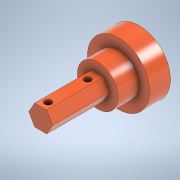
# Autodesk Inventor part: jigForHexBushingForConnectorPiece
Saved by Autodesk Inventor 2022.1 (Build 261234000, 234)
## iProperties
Created: 2020-11-16
Part Number: jigForHexBushingForConnectorPiece
Material: PC/ABS Plastic
Document SubType Name: Modeling
Designer: robst
Density: 0.357273 g/cm^3
Appearance: Smooth - Light Orange
Author: robst
Autodesk Inventor part; units mm, degrees
ref_plane "YZ Plane" through (0, 0, 0) normal (1, 0, 0) x (0, 1, 0)
ref_plane "XZ Plane" through (0, 0, 0) normal (0, 1, 0) x (-1, 0, 0)
ref_plane "XY Plane" through (0, 0, 0) normal (0, 0, 1) x (1, 0, 0)
sketch "Sketch1" plane through (0, 0, 0) normal (0, 0, 1) x (1, 0, 0)
  line L0 (7.3323, 0) -> (3.6662, -6.35)
  line L1 (3.6662, -6.35) -> (-3.6662, -6.35)
  line L2 (-3.6662, -6.35) -> (-7.3323, 0)
  line L3 (-7.3323, 0) -> (-3.6662, 6.35)
  line L4 (-3.6662, 6.35) -> (3.6662, 6.35)
  line L5 (3.6662, 6.35) -> (7.3323, 0)
  point P0 (0, 0)
  point P1 (0, 0)
  dimension "d0" = 12.7
  constraints: 12 end point, 1 coincident, 1 horizontal, 13 other
  measures "d0" distance between parallel lines of L1 L4
extrude "Extrusion1" add sketch "Sketch1" along normal mid plane 34.925
sketch "Sketch2" plane through (0, 0, -17.4625) normal (0, 0, -1) x (-1, 0, 0)
  circle A0 centre (0, 0) radius 12.5095
  dimension "d3" = 25.019
  constraints: 1 centre point, 1 coincident
  measures "d3" diameter of A0
extrude "Extrusion2" add sketch "Sketch2" along normal blind 12.7
sketch "Sketch3" plane through (0, 0, -30.1625) normal (0, 0, -1) x (-1, 0, 0)
  circle A0 centre (0, 0) radius 19.05
  dimension "d6" = 38.1
  constraints: 1 centre point, 1 coincident
  measures "d6" diameter of A0
extrude "Extrusion3" add sketch "Sketch3" along normal blind 12.7
sketch "Sketch4" plane through (0, 0, -42.8625) normal (0, 0, -1) x (-1, 0, 0)
  circle A0 centre (0, 0) radius 16.51 construction
  line L0 (-14.4198, 2.5806) -> (-14.4677, 2.1014)
  line L1 (-14.4677, 2.1014) -> (-16.0898, 2.2636)
  spline S0 degree 2 poles (-16.0898, 2.2636) (-16.2865, 2.2832) (-16.6281, 2.2802) (-16.735, 2.235) knots 0 0 0 1 2 2 2
  spline S1 degree 2 poles (-16.735, 2.235) (-16.8484, 2.1874) (-16.9737, 1.9889) (-16.9915, 1.8107) knots 0 0 0 1 2 2 2
  spline S2 degree 2 poles (-16.9915, 1.8107) (-17.0093, 1.6325) (-16.8566, 1.2356) (-16.7212, 1.039) knots 0 0 0 1 2 2 2
  line L2 (-16.7212, 1.039) -> (-14.5952, 0.8264)
  line L3 (-14.5952, 0.8264) -> (-14.6431, 0.3472)
  line L4 (-14.6431, 0.3472) -> (-18.6032, 0.7431)
  line L5 (-18.6032, 0.7431) -> (-18.5553, 1.2224)
  line L6 (-18.5553, 1.2224) -> (-17.1236, 1.0792)
  spline S3 degree 2 poles (-17.1236, 1.0792) (-17.2957, 1.3137) (-17.457, 1.7487) (-17.4336, 1.9822) knots 0 0 0 1 2 2 2
  spline S4 degree 2 poles (-17.4336, 1.9822) (-17.3918, 2.4) (-16.7915, 2.8178) (-16.2662, 2.7653) knots 0 0 0 1 2 2 2
  line L7 (-16.2662, 2.7653) -> (-14.4198, 2.5806)
  spline S5 degree 2 poles (-13.8575, 4.4081) (-14.0557, 3.752) (-15.0096, 3.2532) (-15.6893, 3.4586) knots 0 0 0 1 2 2 2
  spline S6 degree 2 poles (-15.6893, 3.4586) (-16.3573, 3.6604) (-16.9377, 4.6002) (-16.7672, 5.1647) knots 0 0 0 1 2 2 2
  spline S7 degree 2 poles (-16.7672, 5.1647) (-16.6904, 5.4189) (-16.4238, 5.7673) (-16.2234, 5.8648) knots 0 0 0 1 2 2 2
  spline S8 degree 2 poles (-16.2234, 5.8648) (-16.0221, 5.9653) (-15.5226, 5.9853) (-15.1945, 5.8861) knots 0 0 0 1 2 2 2
  line L8 (-15.1945, 5.8861) -> (-14.9433, 5.8102)
  line L9 (-14.9433, 5.8102) -> (-15.5157, 3.9157)
  spline S9 degree 2 poles (-15.5157, 3.9157) (-15.0399, 3.7719) (-14.3898, 4.098) (-14.2612, 4.5236) knots 0 0 0 1 2 2 2
  spline S10 degree 2 poles (-14.2612, 4.5236) (-14.2157, 4.6744) (-14.1952, 4.9875) (-14.2127, 5.1218) knots 0 0 0 1 2 2 2
  spline S11 degree 2 poles (-14.2127, 5.1218) (-14.2343, 5.2638) (-14.286, 5.4665) (-14.3163, 5.5369) knots 0 0 0 1 2 2 2
  line L10 (-14.3163, 5.5369) -> (-14.3083, 5.5635)
  line L11 (-14.3083, 5.5635) -> (-13.8058, 5.4117)
  spline S12 degree 2 poles (-13.8058, 5.4117) (-13.7974, 5.3221) (-13.7761, 5.0511) (-13.778, 4.9485) knots 0 0 0 1 2 2 2
  spline S13 degree 2 poles (-13.778, 4.9485) (-13.7798, 4.8039) (-13.8075, 4.5736) (-13.8575, 4.4081) knots 0 0 0 1 2 2 2
  spline S14 degree 2 poles (-15.4307, 5.4673) (-15.6187, 5.5176) (-15.9139, 5.5229) (-16.0278, 5.4767) knots 0 0 0 1 2 2 2
  spline S15 degree 2 poles (-16.0278, 5.4767) (-16.1554, 5.4282) (-16.3406, 5.21) (-16.3969, 5.0238) knots 0 0 0 1 2 2 2
  spline S16 degree 2 poles (-16.3969, 5.0238) (-16.4523, 4.8406) (-16.4206, 4.5504) (-16.3464, 4.4118) knots 0 0 0 1 2 2 2
  spline S17 degree 2 poles (-16.3464, 4.4118) (-16.2683, 4.2753) (-16.0374, 4.0895) (-15.8674, 4.022) knots 0 0 0 1 2 2 2
  line L12 (-15.8674, 4.022) -> (-15.4307, 5.4673)
  line L13 (-12.3977, 7.8243) -> (-12.668, 7.3002)
  line L14 (-12.668, 7.3002) -> (-13.9414, 7.1752)
  line L15 (-13.9414, 7.1752) -> (-13.3133, 6.0489)
  line L16 (-13.3133, 6.0489) -> (-13.5637, 5.5632)
  line L17 (-13.5637, 5.5632) -> (-14.3691, 7.0936)
  line L18 (-14.3691, 7.0936) -> (-16.1006, 6.8818)
  line L19 (-16.1006, 6.8818) -> (-15.8303, 7.4059)
  line L20 (-15.8303, 7.4059) -> (-14.5666, 7.5324)
  line L21 (-14.5666, 7.5324) -> (-15.1893, 8.649)
  line L22 (-15.1893, 8.649) -> (-14.9388, 9.1347)
  line L23 (-14.9388, 9.1347) -> (-14.1361, 7.6126)
  line L24 (-14.1361, 7.6126) -> (-12.3977, 7.8243)
  spline S18 degree 2 poles (-11.4795, 10.9139) (-11.2568, 10.7375) (-11.0498, 10.2978) (-11.0496, 10.0692) knots 0 0 0 1 2 2 2
  spline S19 degree 2 poles (-11.0496, 10.0692) (-11.0532, 9.7963) (-11.2467, 9.3233) (-11.4882, 9.0183) knots 0 0 0 1 2 2 2
  line L25 (-11.4882, 9.0183) -> (-12.167, 8.1616)
  line L26 (-12.167, 8.1616) -> (-15.1534, 10.5275)
  line L27 (-15.1534, 10.5275) -> (-14.5264, 11.3189)
  spline S20 degree 2 poles (-14.5264, 11.3189) (-14.2734, 11.6383) (-13.9792, 11.9252) (-13.7843, 12.0071) knots 0 0 0 1 2 2 2
  spline S21 degree 2 poles (-13.7843, 12.0071) (-13.5711, 12.1022) (-13.1758, 12.0293) (-12.9871, 11.8798) knots 0 0 0 1 2 2 2
  spline S22 degree 2 poles (-12.9871, 11.8798) (-12.7765, 11.713) (-12.6189, 11.2257) (-12.6798, 10.9549) knots 0 0 0 1 2 2 2
  line L28 (-12.6798, 10.9549) -> (-12.6653, 10.9434)
  spline S23 degree 2 poles (-12.6653, 10.9434) (-12.3818, 11.1521) (-11.765, 11.1401) (-11.4795, 10.9139) knots 0 0 0 1 2 2 2
  spline S24 degree 2 poles (-11.7904, 10.4866) (-11.9598, 10.6208) (-12.2543, 10.6966) (-12.4467, 10.6127) knots 0 0 0 1 2 2 2
  spline S25 degree 2 poles (-12.4467, 10.6127) (-12.5699, 10.5567) (-12.7753, 10.357) (-12.9383, 10.1513) knots 0 0 0 1 2 2 2
  line L29 (-12.9383, 10.1513) -> (-13.2949, 9.7012)
  line L30 (-13.2949, 9.7012) -> (-12.1913, 8.8269)
  line L31 (-12.1913, 8.8269) -> (-11.9363, 9.1488)
  spline S26 degree 2 poles (-11.9363, 9.1488) (-11.7293, 9.4102) (-11.54, 9.7486) (-11.5254, 9.9261) knots 0 0 0 1 2 2 2
  spline S27 degree 2 poles (-11.5254, 9.9261) (-11.517, 10.1007) (-11.6331, 10.362) (-11.7904, 10.4866) knots 0 0 0 1 2 2 2
  spline S28 degree 2 poles (-13.2592, 11.4218) (-13.3657, 11.5062) (-13.583, 11.5601) (-13.6922, 11.5167) knots 0 0 0 1 2 2 2
  spline S29 degree 2 poles (-13.6922, 11.5167) (-13.8222, 11.4621) (-14.0323, 11.2465) (-14.1991, 11.0359) knots 0 0 0 1 2 2 2
  line L32 (-14.1991, 11.0359) -> (-14.5001, 10.656)
  line L33 (-14.5001, 10.656) -> (-13.6265, 9.9638)
  line L34 (-13.6265, 9.9638) -> (-13.2699, 10.414)
  spline S30 degree 2 poles (-13.2699, 10.414) (-13.1222, 10.6003) (-13.021, 10.8077) (-13.0067, 10.95) knots 0 0 0 1 2 2 2
  spline S31 degree 2 poles (-13.0067, 10.95) (-12.992, 11.088) (-13.1189, 11.3106) (-13.2592, 11.4218) knots 0 0 0 1 2 2 2
  line L35 (-8.5093, 11.9219) -> (-8.879, 11.6132)
  line L36 (-8.879, 11.6132) -> (-9.0809, 11.8549)
  spline S32 degree 2 poles (-9.0809, 11.8549) (-9.1268, 11.5631) (-9.3038, 11.1537) (-9.4934, 10.9954) knots 0 0 0 1 2 2 2
  spline S33 degree 2 poles (-9.4934, 10.9954) (-9.6356, 10.8767) (-9.9683, 10.7597) (-10.1459, 10.7844) knots 0 0 0 1 2 2 2
  spline S34 degree 2 poles (-10.1459, 10.7844) (-10.3257, 10.8071) (-10.6893, 11.0304) (-10.8753, 11.2532) knots 0 0 0 1 2 2 2
  line L37 (-10.8753, 11.2532) -> (-12.0649, 12.6774)
  line L38 (-12.0649, 12.6774) -> (-11.6952, 12.9861)
  line L39 (-11.6952, 12.9861) -> (-10.6502, 11.7349)
  spline S35 degree 2 poles (-10.6502, 11.7349) (-10.5037, 11.5596) (-10.2856, 11.3515) (-10.1694, 11.3038) knots 0 0 0 1 2 2 2
  spline S36 degree 2 poles (-10.1694, 11.3038) (-10.0531, 11.2561) (-9.8337, 11.3065) (-9.6892, 11.4273) knots 0 0 0 1 2 2 2
  spline S37 degree 2 poles (-9.6892, 11.4273) (-9.5541, 11.5401) (-9.3771, 11.9494) (-9.3421, 12.1677) knots 0 0 0 1 2 2 2
  line L40 (-9.3421, 12.1677) -> (-10.7118, 13.8075)
  line L41 (-10.7118, 13.8075) -> (-10.3421, 14.1163)
  line L42 (-10.3421, 14.1163) -> (-8.5093, 11.9219)
  spline S38 degree 2 poles (-7.2187, 12.6182) (-7.4684, 12.4765) (-7.9769, 12.3653) (-8.1619, 12.3597) knots 0 0 0 1 2 2 2
  line L43 (-8.1619, 12.3597) -> (-8.4286, 12.8296)
  line L44 (-8.4286, 12.8296) -> (-8.4071, 12.8417)
  spline S39 degree 2 poles (-8.4071, 12.8417) (-8.3291, 12.8293) (-8.1261, 12.8096) (-7.9733, 12.8218) knots 0 0 0 1 2 2 2
  spline S40 degree 2 poles (-7.9733, 12.8218) (-7.8396, 12.8302) (-7.5392, 12.9014) (-7.4023, 12.9791) knots 0 0 0 1 2 2 2
  spline S41 degree 2 poles (-7.4023, 12.9791) (-7.3029, 13.0355) (-7.1006, 13.2107) (-7.0682, 13.2788) knots 0 0 0 1 2 2 2
  spline S42 degree 2 poles (-7.0682, 13.2788) (-7.0193, 13.374) (-7.0151, 13.5291) (-7.0821, 13.6472) knots 0 0 0 1 2 2 2
  spline S43 degree 2 poles (-7.0821, 13.6472) (-7.166, 13.7949) (-7.414, 13.8565) (-7.6497, 13.7901) knots 0 0 0 1 2 2 2
  spline S44 degree 2 poles (-7.6497, 13.7901) (-7.7409, 13.7632) (-8.0291, 13.6706) (-8.156, 13.6376) knots 0 0 0 1 2 2 2
  spline S45 degree 2 poles (-8.156, 13.6376) (-8.4879, 13.5593) (-8.9407, 13.7566) (-9.0794, 14.0009) knots 0 0 0 1 2 2 2
  spline S46 degree 2 poles (-9.0794, 14.0009) (-9.2715, 14.3392) (-9.0034, 15.0489) (-8.5845, 15.2867) knots 0 0 0 1 2 2 2
  spline S47 degree 2 poles (-8.5845, 15.2867) (-8.3778, 15.4041) (-7.901, 15.5398) (-7.7145, 15.5428) knots 0 0 0 1 2 2 2
  line L45 (-7.7145, 15.5428) -> (-7.4599, 15.0944)
  line L46 (-7.4599, 15.0944) -> (-7.4814, 15.0822)
  spline S48 degree 2 poles (-7.4814, 15.0822) (-7.7157, 15.1196) (-8.1915, 15.0447) (-8.3929, 14.9304) knots 0 0 0 1 2 2 2
  spline S49 degree 2 poles (-8.3929, 14.9304) (-8.5996, 14.813) (-8.7852, 14.4769) (-8.6861, 14.3024) knots 0 0 0 1 2 2 2
  spline S50 degree 2 poles (-8.6861, 14.3024) (-8.5961, 14.144) (-8.3401, 14.087) (-8.1247, 14.1453) knots 0 0 0 1 2 2 2
  spline S51 degree 2 poles (-8.1247, 14.1453) (-8.0197, 14.173) (-7.7613, 14.2557) (-7.6184, 14.2979) knots 0 0 0 1 2 2 2
  spline S52 degree 2 poles (-7.6184, 14.2979) (-7.3049, 14.3835) (-6.8442, 14.2225) (-6.6872, 13.946) knots 0 0 0 1 2 2 2
  spline S53 degree 2 poles (-6.6872, 13.946) (-6.5958, 13.7849) (-6.5604, 13.4286) (-6.6245, 13.2538) knots 0 0 0 1 2 2 2
  spline S54 degree 2 poles (-6.6245, 13.2538) (-6.6935, 13.069) (-6.9636, 12.763) (-7.2187, 12.6182) knots 0 0 0 1 2 2 2
  line L47 (-3.7576, 14.1588) -> (-4.2122, 13.9996)
  line L48 (-4.2122, 13.9996) -> (-4.751, 15.5382)
  spline S55 degree 2 poles (-4.751, 15.5382) (-4.8163, 15.7247) (-4.9635, 16.033) (-5.0496, 16.1108) knots 0 0 0 1 2 2 2
  spline S56 degree 2 poles (-5.0496, 16.1108) (-5.1407, 16.1934) (-5.3736, 16.223) (-5.5426, 16.1639) knots 0 0 0 1 2 2 2
  spline S57 degree 2 poles (-5.5426, 16.1639) (-5.7116, 16.1047) (-6.0068, 15.7985) (-6.1277, 15.5926) knots 0 0 0 1 2 2 2
  line L49 (-6.1277, 15.5926) -> (-5.4215, 13.5761)
  line L50 (-5.4215, 13.5761) -> (-5.8761, 13.4169)
  line L51 (-5.8761, 13.4169) -> (-7.1915, 17.1731)
  line L52 (-7.1915, 17.1731) -> (-6.7369, 17.3322)
  line L53 (-6.7369, 17.3322) -> (-6.2613, 15.9743)
  spline S58 degree 2 poles (-6.2613, 15.9743) (-6.1216, 16.2293) (-5.7956, 16.5594) (-5.5741, 16.637) knots 0 0 0 1 2 2 2
  spline S59 degree 2 poles (-5.5741, 16.637) (-5.1778, 16.7757) (-4.5454, 16.4084) (-4.3709, 15.9101) knots 0 0 0 1 2 2 2
  line L54 (-4.3709, 15.9101) -> (-3.7576, 14.1588)
  line L55 (-2.6108, 14.3718) -> (-3.0832, 14.2779)
  line L56 (-3.0832, 14.2779) -> (-3.6405, 17.0821)
  line L57 (-3.6405, 17.0821) -> (-3.1681, 17.176)
  line L58 (-3.1681, 17.176) -> (-2.6108, 14.3718)
  line L59 (-3.2275, 17.6489) -> (-3.7635, 17.5424)
  line L60 (-3.7635, 17.5424) -> (-3.861, 18.033)
  line L61 (-3.861, 18.033) -> (-3.325, 18.1395)
  line L62 (-3.325, 18.1395) -> (-3.2275, 17.6489)
  line L63 (0.3206, 14.6454) -> (-0.1603, 14.6186)
  line L64 (-0.1603, 14.6186) -> (-0.2508, 16.2463)
  spline S60 degree 2 poles (-0.2508, 16.2463) (-0.2617, 16.4436) (-0.3176, 16.7807) (-0.3787, 16.8793) knots 0 0 0 1 2 2 2
  spline S61 degree 2 poles (-0.3787, 16.8793) (-0.4433, 16.984) (-0.6588, 17.0771) (-0.8376, 17.0672) knots 0 0 0 1 2 2 2
  spline S62 degree 2 poles (-0.8376, 17.0672) (-1.0164, 17.0572) (-1.3849, 16.845) (-1.5582, 16.6808) knots 0 0 0 1 2 2 2
  line L65 (-1.5582, 16.6808) -> (-1.4396, 14.5475)
  line L66 (-1.4396, 14.5475) -> (-1.9205, 14.5208)
  line L67 (-1.9205, 14.5208) -> (-2.0792, 17.3754)
  line L68 (-2.0792, 17.3754) -> (-1.5983, 17.4022)
  line L69 (-1.5983, 17.4022) -> (-1.5807, 17.0846)
  spline S63 degree 2 poles (-1.5807, 17.0846) (-1.3757, 17.2908) (-0.9708, 17.5174) (-0.7365, 17.5305) knots 0 0 0 1 2 2 2
  spline S64 degree 2 poles (-0.7365, 17.5305) (-0.3173, 17.5538) (0.1883, 17.0253) (0.2176, 16.4981) knots 0 0 0 1 2 2 2
  line L70 (0.2176, 16.4981) -> (0.3206, 14.6454)
  spline S65 degree 2 poles (1.0284, 14.1458) (1.0743, 14.1174) (1.251, 14.0233) (1.3662, 13.9787) knots 0 0 0 1 2 2 2
  spline S66 degree 2 poles (1.3662, 13.9787) (1.4928, 13.9261) (1.7102, 13.8543) (1.8416, 13.8354) knots 0 0 0 1 2 2 2
  spline S67 degree 2 poles (1.8416, 13.8354) (2.0616, 13.8037) (2.3839, 13.8759) (2.4844, 13.9674) knots 0 0 0 1 2 2 2
  spline S68 degree 2 poles (2.4844, 13.9674) (2.5819, 14.0595) (2.6852, 14.3222) (2.7103, 14.4964) knots 0 0 0 1 2 2 2
  line L71 (2.7103, 14.4964) -> (2.7459, 14.744)
  spline S69 degree 2 poles (2.7459, 14.744) (2.5292, 14.6036) (2.1366, 14.4979) (1.8585, 14.5379) knots 0 0 0 1 2 2 2
  spline S70 degree 2 poles (1.8585, 14.5379) (1.3756, 14.6074) (0.9075, 15.4078) (1.0047, 16.0832) knots 0 0 0 1 2 2 2
  spline S71 degree 2 poles (1.0047, 16.0832) (1.0553, 16.4347) (1.3322, 16.95) (1.525, 17.1188) knots 0 0 0 1 2 2 2
  spline S72 degree 2 poles (1.525, 17.1188) (1.7098, 17.2763) (2.1754, 17.412) (2.4077, 17.3786) knots 0 0 0 1 2 2 2
  spline S73 degree 2 poles (2.4077, 17.3786) (2.6277, 17.3469) (2.9336, 17.1968) (3.082, 17.0788) knots 0 0 0 1 2 2 2
  line L72 (3.082, 17.0788) -> (3.1266, 17.194)
  line L73 (3.1266, 17.194) -> (3.5759, 17.1293)
  line L74 (3.5759, 17.1293) -> (3.2152, 14.6234)
  spline S74 degree 2 poles (3.2152, 14.6234) (3.1114, 13.9022) (2.3881, 13.32) (1.7433, 13.4128) knots 0 0 0 1 2 2 2
  spline S75 degree 2 poles (1.7433, 13.4128) (1.5355, 13.4427) (1.1112, 13.5724) (0.9327, 13.6543) knots 0 0 0 1 2 2 2
  line L75 (0.9327, 13.6543) -> (1.004, 14.1493)
  line L76 (1.004, 14.1493) -> (1.0284, 14.1458)
  line L77 (2.8022, 15.1351) -> (3.0261, 16.6906)
  spline S76 degree 2 poles (3.0261, 16.6906) (2.8612, 16.8017) (2.5723, 16.9182) (2.4225, 16.9397) knots 0 0 0 1 2 2 2
  spline S77 degree 2 poles (2.4225, 16.9397) (2.0619, 16.9916) (1.5697, 16.5197) (1.498, 16.0216) knots 0 0 0 1 2 2 2
  spline S78 degree 2 poles (1.498, 16.0216) (1.4303, 15.5509) (1.6743, 15.0136) (2.0288, 14.9626) knots 0 0 0 1 2 2 2
  spline S79 degree 2 poles (2.0288, 14.9626) (2.2152, 14.9358) (2.6275, 15.0262) (2.8022, 15.1351) knots 0 0 0 1 2 2 2
  line L78 (7.133, 16.5384) -> (5.4593, 17.1212)
  line L79 (5.4593, 17.1212) -> (5.106, 16.1065)
  line L80 (5.106, 16.1065) -> (6.7097, 15.5481)
  line L81 (6.7097, 15.5481) -> (6.5615, 15.1224)
  line L82 (6.5615, 15.1224) -> (4.9577, 15.6807)
  line L83 (4.9577, 15.6807) -> (4.3547, 13.9487)
  line L84 (4.3547, 13.9487) -> (3.8765, 14.1152)
  line L85 (3.8765, 14.1152) -> (5.1293, 17.7134)
  line L86 (5.1293, 17.7134) -> (7.2812, 16.9641)
  line L87 (7.2812, 16.9641) -> (7.133, 16.5384)
  spline S80 degree 2 poles (9.1463, 13.2318) (8.7839, 12.6068) (7.7881, 12.2741) (7.2859, 12.5652) knots 0 0 0 1 2 2 2
  spline S81 degree 2 poles (7.2859, 12.5652) (6.7703, 12.864) (6.5873, 13.9088) (6.9372, 14.5124) knots 0 0 0 1 2 2 2
  spline S82 degree 2 poles (6.9372, 14.5124) (7.2965, 15.1321) (8.3035, 15.4656) (8.8003, 15.1776) knots 0 0 0 1 2 2 2
  spline S83 degree 2 poles (8.8003, 15.1776) (9.3025, 14.8864) (9.5071, 13.8542) (9.1463, 13.2318) knots 0 0 0 1 2 2 2
  spline S84 degree 2 poles (8.7162, 13.4811) (8.9949, 13.962) (8.916, 14.6323) (8.5928, 14.8196) knots 0 0 0 1 2 2 2
  spline S85 degree 2 poles (8.5928, 14.8196) (8.2696, 15.007) (7.646, 14.7439) (7.3673, 14.2631) knots 0 0 0 1 2 2 2
  spline S86 degree 2 poles (7.3673, 14.2631) (7.0963, 13.7957) (7.1702, 13.1105) (7.4934, 12.9231) knots 0 0 0 1 2 2 2
  spline S87 degree 2 poles (7.4934, 12.9231) (7.8139, 12.7373) (8.4406, 13.0057) (8.7162, 13.4811) knots 0 0 0 1 2 2 2
  line L88 (11.4605, 12.5201) -> (11.4414, 12.5358)
  spline S88 degree 2 poles (11.4414, 12.5358) (11.4082, 12.583) (11.319, 12.6641) (11.2546, 12.717) knots 0 0 0 1 2 2 2
  spline S89 degree 2 poles (11.2546, 12.717) (11.1042, 12.8403) (10.7005, 12.9519) (10.4611, 12.9326) knots 0 0 0 1 2 2 2
  line L89 (10.4611, 12.9326) -> (9.1745, 11.3643)
  line L90 (9.1745, 11.3643) -> (8.8022, 11.6698)
  line L91 (8.8022, 11.6698) -> (10.6154, 13.8802)
  line L92 (10.6154, 13.8802) -> (10.9878, 13.5747)
  line L93 (10.9878, 13.5747) -> (10.7176, 13.2453)
  spline S90 degree 2 poles (10.7176, 13.2453) (11.0693, 13.2603) (11.4939, 13.1596) (11.6371, 13.0421) knots 0 0 0 1 2 2 2
  spline S91 degree 2 poles (11.6371, 13.0421) (11.6944, 12.9951) (11.7478, 12.9434) (11.7777, 12.9068) knots 0 0 0 1 2 2 2
  line L94 (11.7777, 12.9068) -> (11.4605, 12.5201)
  spline S92 degree 2 poles (11.203, 9.2687) (10.961, 9.5492) (10.7409, 10.1871) (10.781, 10.5235) knots 0 0 0 1 2 2 2
  spline S93 degree 2 poles (10.781, 10.5235) (10.8187, 10.8579) (11.2164, 11.5313) (11.5811, 11.8459) knots 0 0 0 1 2 2 2
  spline S94 degree 2 poles (11.5811, 11.8459) (11.9434, 12.1586) (12.6404, 12.4378) (12.9904, 12.4339) knots 0 0 0 1 2 2 2
  spline S95 degree 2 poles (12.9904, 12.4339) (13.3337, 12.4283) (13.9445, 12.1316) (14.1966, 11.8394) knots 0 0 0 1 2 2 2
  spline S96 degree 2 poles (14.1966, 11.8394) (14.3216, 11.6945) (14.4994, 11.4034) (14.5595, 11.2676) knots 0 0 0 1 2 2 2
  spline S97 degree 2 poles (14.5595, 11.2676) (14.6098, 11.1479) (14.6907, 10.8792) (14.7219, 10.739) knots 0 0 0 1 2 2 2
  line L95 (14.7219, 10.739) -> (14.2591, 10.3396)
  line L96 (14.2591, 10.3396) -> (14.2329, 10.37)
  spline S98 degree 2 poles (14.2329, 10.37) (14.2353, 10.4618) (14.229, 10.7337) (14.1933, 10.9027) knots 0 0 0 1 2 2 2
  spline S99 degree 2 poles (14.1933, 10.9027) (14.1593, 11.065) (14.0125, 11.3911) (13.8673, 11.5594) knots 0 0 0 1 2 2 2
  spline S100 degree 2 poles (13.8673, 11.5594) (13.708, 11.744) (13.2716, 11.9425) (13.0198, 11.9414) knots 0 0 0 1 2 2 2
  spline S101 degree 2 poles (13.0198, 11.9414) (12.7676, 11.9359) (12.2042, 11.6862) (11.926, 11.4462) knots 0 0 0 1 2 2 2
  spline S102 degree 2 poles (11.926, 11.4462) (11.6291, 11.19) (11.3243, 10.6783) (11.284, 10.4274) knots 0 0 0 1 2 2 2
  spline S103 degree 2 poles (11.284, 10.4274) (11.2463, 10.1828) (11.3817, 9.7328) (11.539, 9.5505) knots 0 0 0 1 2 2 2
  spline S104 degree 2 poles (11.539, 9.5505) (11.6822, 9.3845) (12.0081, 9.1722) (12.1637, 9.1148) knots 0 0 0 1 2 2 2
  spline S105 degree 2 poles (12.1637, 9.1148) (12.3152, 9.062) (12.5766, 9.0143) (12.6593, 9.0082) knots 0 0 0 1 2 2 2
  line L97 (12.6593, 9.0082) -> (12.6835, 8.9802)
  line L98 (12.6835, 8.9802) -> (12.2254, 8.5849)
  spline S106 degree 2 poles (12.2254, 8.5849) (12.0982, 8.6424) (11.8712, 8.7401) (11.7309, 8.827) knots 0 0 0 1 2 2 2
  spline S107 degree 2 poles (11.7309, 8.827) (11.5799, 8.917) (11.3523, 9.0957) (11.203, 9.2687) knots 0 0 0 1 2 2 2
  spline S108 degree 2 poles (14.6337, 6.6777) (14.0023, 6.3266) (12.9765, 6.551) (12.6944, 7.0583) knots 0 0 0 1 2 2 2
  spline S109 degree 2 poles (12.6944, 7.0583) (12.4048, 7.5791) (12.7828, 8.57) (13.3926, 8.9092) knots 0 0 0 1 2 2 2
  spline S110 degree 2 poles (13.3926, 8.9092) (14.0186, 9.2574) (15.0542, 9.0278) (15.3334, 8.5259) knots 0 0 0 1 2 2 2
  spline S111 degree 2 poles (15.3334, 8.5259) (15.6155, 8.0187) (15.2624, 7.0274) (14.6337, 6.6777) knots 0 0 0 1 2 2 2
  spline S112 degree 2 poles (14.3921, 7.1121) (14.8777, 7.3823) (15.1534, 7.9983) (14.9718, 8.3248) knots 0 0 0 1 2 2 2
  spline S113 degree 2 poles (14.9718, 8.3248) (14.7902, 8.6513) (14.1199, 8.7449) (13.6342, 8.4748) knots 0 0 0 1 2 2 2
  spline S114 degree 2 poles (13.6342, 8.4748) (13.162, 8.2122) (12.8744, 7.5859) (13.056, 7.2594) knots 0 0 0 1 2 2 2
  spline S115 degree 2 poles (13.056, 7.2594) (13.2361, 6.9356) (13.9118, 6.845) (14.3921, 7.1121) knots 0 0 0 1 2 2 2
  line L99 (14.2516, 3.3884) -> (14.1043, 3.8469)
  line L100 (14.1043, 3.8469) -> (15.6564, 4.3456)
  spline S116 degree 2 poles (15.6564, 4.3456) (15.8445, 4.406) (16.1565, 4.5452) (16.2365, 4.6292) knots 0 0 0 1 2 2 2
  spline S117 degree 2 poles (16.2365, 4.6292) (16.3215, 4.7181) (16.3572, 4.9501) (16.3024, 5.1206) knots 0 0 0 1 2 2 2
  spline S118 degree 2 poles (16.3024, 5.1206) (16.2477, 5.2911) (15.9493, 5.5941) (15.7466, 5.7204) knots 0 0 0 1 2 2 2
  line L101 (15.7466, 5.7204) -> (13.7124, 5.0669)
  line L102 (13.7124, 5.0669) -> (13.5651, 5.5254)
  line L103 (13.5651, 5.5254) -> (16.2871, 6.3999)
  line L104 (16.2871, 6.3999) -> (16.4344, 5.9413)
  line L105 (16.4344, 5.9413) -> (16.1316, 5.8441)
  spline S119 degree 2 poles (16.1316, 5.8441) (16.3829, 5.6978) (16.7044, 5.3633) (16.7762, 5.1399) knots 0 0 0 1 2 2 2
  spline S120 degree 2 poles (16.7762, 5.1399) (16.9046, 4.7401) (16.521, 4.1174) (16.0183, 3.9559) knots 0 0 0 1 2 2 2
  line L106 (16.0183, 3.9559) -> (14.2516, 3.3884)
  line L107 (14.6404, 0.4994) -> (14.5868, 0.978)
  line L108 (14.5868, 0.978) -> (16.2069, 1.1595)
  spline S121 degree 2 poles (16.2069, 1.1595) (16.4032, 1.1815) (16.7366, 1.2561) (16.8317, 1.3227) knots 0 0 0 1 2 2 2
  spline S122 degree 2 poles (16.8317, 1.3227) (16.9326, 1.393) (17.0135, 1.6133) (16.9936, 1.7913) knots 0 0 0 1 2 2 2
  spline S123 degree 2 poles (16.9936, 1.7913) (16.9737, 1.9692) (16.7411, 2.3253) (16.5675, 2.4892) knots 0 0 0 1 2 2 2
  line L109 (16.5675, 2.4892) -> (14.4442, 2.2514)
  line L110 (14.4442, 2.2514) -> (14.3906, 2.7301)
  line L111 (14.3906, 2.7301) -> (17.2318, 3.0483)
  line L112 (17.2318, 3.0483) -> (17.2854, 2.5696)
  line L113 (17.2854, 2.5696) -> (16.9694, 2.5342)
  spline S124 degree 2 poles (16.9694, 2.5342) (17.1868, 2.3411) (17.4357, 1.9495) (17.4618, 1.7163) knots 0 0 0 1 2 2 2
  spline S125 degree 2 poles (17.4618, 1.7163) (17.5085, 1.299) (17.0091, 0.7647) (16.4844, 0.7059) knots 0 0 0 1 2 2 2
  line L114 (16.4844, 0.7059) -> (14.6404, 0.4994)
  spline S126 degree 2 poles (14.4736, -1.4053) (14.5299, -0.7222) (15.358, -0.0346) (16.0658, -0.0929) knots 0 0 0 1 2 2 2
  spline S127 degree 2 poles (16.0658, -0.0929) (16.7612, -0.1502) (17.5257, -0.9475) (17.4773, -1.5352) knots 0 0 0 1 2 2 2
  spline S128 degree 2 poles (17.4773, -1.5352) (17.4555, -1.7998) (17.2679, -2.1964) (17.0924, -2.3337) knots 0 0 0 1 2 2 2
  spline S129 degree 2 poles (17.0924, -2.3337) (16.9166, -2.4742) (16.4323, -2.5984) (16.0908, -2.5703) knots 0 0 0 1 2 2 2
  line L115 (16.0908, -2.5703) -> (15.8292, -2.5487)
  line L116 (15.8292, -2.5487) -> (15.9918, -0.5763)
  spline S130 degree 2 poles (15.9918, -0.5763) (15.4964, -0.5355) (14.9292, -0.9906) (14.8926, -1.4337) knots 0 0 0 1 2 2 2
  spline S131 degree 2 poles (14.8926, -1.4337) (14.8797, -1.5906) (14.9253, -1.9011) (14.9706, -2.0287) knots 0 0 0 1 2 2 2
  spline S132 degree 2 poles (14.9706, -2.0287) (15.0215, -2.163) (15.1145, -2.3504) (15.1589, -2.4129) knots 0 0 0 1 2 2 2
  line L117 (15.1589, -2.4129) -> (15.1566, -2.4406)
  line L118 (15.1566, -2.4406) -> (14.6335, -2.3975)
  spline S133 degree 2 poles (14.6335, -2.3975) (14.6065, -2.3116) (14.5288, -2.0512) (14.5092, -1.9504) knots 0 0 0 1 2 2 2
  spline S134 degree 2 poles (14.5092, -1.9504) (14.4807, -1.8086) (14.4594, -1.5776) (14.4736, -1.4053) knots 0 0 0 1 2 2 2
  spline S135 degree 2 poles (16.234, -2.1112) (16.4283, -2.121) (16.718, -2.0643) (16.8198, -1.9953) knots 0 0 0 1 2 2 2
  spline S136 degree 2 poles (16.8198, -1.9953) (16.9343, -1.9211) (17.0697, -1.6689) (17.0857, -1.475) knots 0 0 0 1 2 2 2
  spline S137 degree 2 poles (17.0857, -1.475) (17.1014, -1.2843) (17.0096, -1.0072) (16.908, -0.8873) knots 0 0 0 1 2 2 2
  spline S138 degree 2 poles (16.908, -0.8873) (16.803, -0.7702) (16.5383, -0.6368) (16.358, -0.6065) knots 0 0 0 1 2 2 2
  line L119 (16.358, -0.6065) -> (16.234, -2.1112)
  spline S139 degree 2 poles (13.9847, -3.9902) (14.0606, -3.7036) (14.3624, -3.2757) (14.5865, -3.153) knots 0 0 0 1 2 2 2
  spline S140 degree 2 poles (14.5865, -3.153) (14.8077, -3.0296) (15.4007, -2.9854) (15.7648, -3.0819) knots 0 0 0 1 2 2 2
  spline S141 degree 2 poles (15.7648, -3.0819) (16.1289, -3.1783) (16.6088, -3.513) (16.7444, -3.7246) knots 0 0 0 1 2 2 2
  spline S142 degree 2 poles (16.7444, -3.7246) (16.8829, -3.937) (16.9481, -4.4749) (16.8738, -4.7554) knots 0 0 0 1 2 2 2
  spline S143 degree 2 poles (16.8738, -4.7554) (16.8137, -4.9822) (16.5731, -5.3721) (16.446, -5.5141) knots 0 0 0 1 2 2 2
  line L120 (16.446, -5.5141) -> (15.9237, -5.3757)
  line L121 (15.9237, -5.3757) -> (15.9308, -5.3489)
  spline S144 degree 2 poles (15.9308, -5.3489) (15.9861, -5.3092) (16.1346, -5.1825) (16.2206, -5.0871) knots 0 0 0 1 2 2 2
  spline S145 degree 2 poles (16.2206, -5.0871) (16.2944, -5.0012) (16.4386, -4.7583) (16.4702, -4.6389) knots 0 0 0 1 2 2 2
  spline S146 degree 2 poles (16.4702, -4.6389) (16.5659, -4.2778) (16.1359, -3.6944) (15.6375, -3.5624) knots 0 0 0 1 2 2 2
  spline S147 degree 2 poles (15.6375, -3.5624) (15.151, -3.4335) (14.4926, -3.7127) (14.393, -4.0887) knots 0 0 0 1 2 2 2
  spline S148 degree 2 poles (14.393, -4.0887) (14.3329, -4.3155) (14.4118, -4.7772) (14.5162, -4.9741) knots 0 0 0 1 2 2 2
  line L122 (14.5162, -4.9741) -> (14.509, -5.001)
  line L123 (14.509, -5.001) -> (13.9867, -4.8627)
  spline S149 degree 2 poles (13.9867, -4.8627) (13.9721, -4.7853) (13.9349, -4.5519) (13.9361, -4.4628) knots 0 0 0 1 2 2 2
  spline S150 degree 2 poles (13.9361, -4.4628) (13.932, -4.3339) (13.9459, -4.1364) (13.9847, -3.9902) knots 0 0 0 1 2 2 2
  spline S151 degree 2 poles (13.261, -5.9954) (13.4142, -5.6344) (13.9989, -5.403) (14.4451, -5.5924) knots 0 0 0 1 2 2 2
  line L124 (14.4451, -5.5924) -> (15.903, -6.2114)
  line L125 (15.903, -6.2114) -> (16.0297, -5.913)
  line L126 (16.0297, -5.913) -> (16.3963, -6.0686)
  line L127 (16.3963, -6.0686) -> (16.2696, -6.367)
  line L128 (16.2696, -6.367) -> (17.0256, -6.6879)
  line L129 (17.0256, -6.6879) -> (16.8374, -7.1313)
  line L130 (16.8374, -7.1313) -> (16.0814, -6.8104)
  line L131 (16.0814, -6.8104) -> (15.7351, -7.626)
  line L132 (15.7351, -7.626) -> (15.3685, -7.4704)
  line L133 (15.3685, -7.4704) -> (15.7148, -6.6547)
  line L134 (15.7148, -6.6547) -> (14.4615, -6.1226)
  spline S152 degree 2 poles (14.4615, -6.1226) (14.2625, -6.0382) (14.0377, -5.9595) (13.9234, -5.968) knots 0 0 0 1 2 2 2
  spline S153 degree 2 poles (13.9234, -5.968) (13.8241, -5.9728) (13.6656, -6.1168) (13.6005, -6.2703) knots 0 0 0 1 2 2 2
  spline S154 degree 2 poles (13.6005, -6.2703) (13.5546, -6.3783) (13.5343, -6.6078) (13.5349, -6.6618) knots 0 0 0 1 2 2 2
  line L135 (13.5349, -6.6618) -> (13.5241, -6.6873)
  line L136 (13.5241, -6.6873) -> (13.1262, -6.5184)
  spline S155 degree 2 poles (13.1262, -6.5184) (13.1452, -6.3789) (13.214, -6.1062) (13.261, -5.9954) knots 0 0 0 1 2 2 2
  spline S156 degree 2 poles (12.9217, -9.5795) (12.309, -9.1966) (12.0094, -8.1903) (12.317, -7.698) knots 0 0 0 1 2 2 2
  spline S157 degree 2 poles (12.317, -7.698) (12.6327, -7.1927) (13.683, -7.0443) (14.2747, -7.4141) knots 0 0 0 1 2 2 2
  spline S158 degree 2 poles (14.2747, -7.4141) (14.8822, -7.7936) (15.1821, -8.8111) (14.8778, -9.2981) knots 0 0 0 1 2 2 2
  spline S159 degree 2 poles (14.8778, -9.2981) (14.5702, -9.7904) (13.5318, -9.9607) (12.9217, -9.5795) knots 0 0 0 1 2 2 2
  spline S160 degree 2 poles (13.1851, -9.1579) (13.6564, -9.4524) (14.3289, -9.3957) (14.5269, -9.0789) knots 0 0 0 1 2 2 2
  spline S161 degree 2 poles (14.5269, -9.0789) (14.7249, -8.7621) (14.4826, -8.1301) (14.0113, -7.8356) knots 0 0 0 1 2 2 2
  spline S162 degree 2 poles (14.0113, -7.8356) (13.5531, -7.5493) (12.8658, -7.6004) (12.6678, -7.9173) knots 0 0 0 1 2 2 2
  spline S163 degree 2 poles (12.6678, -7.9173) (12.4715, -8.2315) (12.719, -8.8667) (13.1851, -9.1579) knots 0 0 0 1 2 2 2
  line L137 (12.1337, -11.8688) -> (12.15, -11.8503)
  spline S164 degree 2 poles (12.15, -11.8503) (12.1982, -11.8187) (12.2823, -11.7322) (12.3373, -11.6696) knots 0 0 0 1 2 2 2
  spline S165 degree 2 poles (12.3373, -11.6696) (12.4655, -11.5234) (12.5904, -11.1236) (12.5791, -10.8836) knots 0 0 0 1 2 2 2
  line L138 (12.5791, -10.8836) -> (11.0542, -9.5459)
  line L139 (11.0542, -9.5459) -> (11.3718, -9.1838)
  line L140 (11.3718, -9.1838) -> (13.521, -11.0693)
  line L141 (13.521, -11.0693) -> (13.2034, -11.4314)
  line L142 (13.2034, -11.4314) -> (12.8831, -11.1504)
  spline S166 degree 2 poles (12.8831, -11.1504) (12.8864, -11.5024) (12.7717, -11.9234) (12.6496, -12.0627) knots 0 0 0 1 2 2 2
  spline S167 degree 2 poles (12.6496, -12.0627) (12.6007, -12.1184) (12.5472, -12.17) (12.5097, -12.1987) knots 0 0 0 1 2 2 2
  line L143 (12.5097, -12.1987) -> (12.1337, -11.8688)
  spline S168 degree 2 poles (9.914, -14.2008) (9.7572, -14.0099) (9.6111, -13.5546) (9.6348, -13.3354) knots 0 0 0 1 2 2 2
  spline S169 degree 2 poles (9.6348, -13.3354) (9.6641, -13.0597) (9.9496, -12.5656) (10.2646, -12.307) knots 0 0 0 1 2 2 2
  line L144 (10.2646, -12.307) -> (10.5963, -12.0347)
  line L145 (10.5963, -12.0347) -> (9.695, -10.937)
  line L146 (9.695, -10.937) -> (10.0864, -10.6157)
  line L147 (10.0864, -10.6157) -> (12.5041, -13.5603)
  line L148 (12.5041, -13.5603) -> (11.7643, -14.1677)
  spline S170 degree 2 poles (11.7643, -14.1677) (11.5019, -14.3832) (11.0638, -14.599) (10.8427, -14.6168) knots 0 0 0 1 2 2 2
  spline S171 degree 2 poles (10.8427, -14.6168) (10.586, -14.6398) (10.1158, -14.4466) (9.914, -14.2008) knots 0 0 0 1 2 2 2
  spline S172 degree 2 poles (10.3122, -13.8539) (10.4376, -14.0066) (10.7268, -14.1447) (10.8929, -14.1281) knots 0 0 0 1 2 2 2
  spline S173 degree 2 poles (10.8929, -14.1281) (11.0369, -14.1137) (11.3262, -13.9601) (11.51, -13.8092) knots 0 0 0 1 2 2 2
  line L149 (11.51, -13.8092) -> (11.8345, -13.5428)
  line L150 (11.8345, -13.5428) -> (10.8706, -12.3687)
  line L151 (10.8706, -12.3687) -> (10.6033, -12.5882)
  spline S174 degree 2 poles (10.6033, -12.5882) (10.3647, -12.7841) (10.1339, -13.1015) (10.1207, -13.28) knots 0 0 0 1 2 2 2
  spline S175 degree 2 poles (10.1207, -13.28) (10.1049, -13.4408) (10.1966, -13.7131) (10.3122, -13.8539) knots 0 0 0 1 2 2 2
  line L152 (7.4014, -12.593) -> (7.8126, -12.3421)
  line L153 (7.8126, -12.3421) -> (9.3017, -14.7827)
  line L154 (9.3017, -14.7827) -> (8.8906, -15.0336)
  line L155 (8.8906, -15.0336) -> (7.4014, -12.593)
  line L156 (9.1092, -15.4572) -> (9.5757, -15.1725)
  line L157 (9.5757, -15.1725) -> (9.8363, -15.5995)
  line L158 (9.8363, -15.5995) -> (9.3698, -15.8841)
  line L159 (9.3698, -15.8841) -> (9.1092, -15.4572)
  spline S176 degree 2 poles (5.6387, -13.404) (6.2666, -13.129) (7.2651, -13.5311) (7.5499, -14.1815) knots 0 0 0 1 2 2 2
  spline S177 degree 2 poles (7.5499, -14.1815) (7.8298, -14.8207) (7.4914, -15.8722) (6.9512, -16.1088) knots 0 0 0 1 2 2 2
  spline S178 degree 2 poles (6.9512, -16.1088) (6.708, -16.2153) (6.2699, -16.2386) (6.0657, -16.1494) knots 0 0 0 1 2 2 2
  spline S179 degree 2 poles (6.0657, -16.1494) (5.8586, -16.0614) (5.5193, -15.6943) (5.3818, -15.3804) knots 0 0 0 1 2 2 2
  line L160 (5.3818, -15.3804) -> (5.2765, -15.14)
  line L161 (5.2765, -15.14) -> (7.0894, -14.3461)
  spline S180 degree 2 poles (7.0894, -14.3461) (6.89, -13.8908) (6.2201, -13.6078) (5.8128, -13.7861) knots 0 0 0 1 2 2 2
  spline S181 degree 2 poles (5.8128, -13.7861) (5.6686, -13.8493) (5.417, -14.0369) (5.3262, -14.1374) knots 0 0 0 1 2 2 2
  spline S182 degree 2 poles (5.3262, -14.1374) (5.2322, -14.246) (5.1115, -14.4168) (5.0776, -14.4856) knots 0 0 0 1 2 2 2
  line L162 (5.0776, -14.4856) -> (5.0521, -14.4967)
  line L163 (5.0521, -14.4967) -> (4.8416, -14.0159)
  spline S183 degree 2 poles (4.8416, -14.0159) (4.9043, -13.9514) (5.0966, -13.7593) (5.176, -13.6942) knots 0 0 0 1 2 2 2
  spline S184 degree 2 poles (5.176, -13.6942) (5.2871, -13.6017) (5.4803, -13.4733) (5.6387, -13.404) knots 0 0 0 1 2 2 2
  spline S185 degree 2 poles (5.8538, -15.2883) (5.9375, -15.464) (6.1249, -15.692) (6.234, -15.7487) knots 0 0 0 1 2 2 2
  spline S186 degree 2 poles (6.234, -15.7487) (6.3538, -15.8143) (6.64, -15.8136) (6.8182, -15.7356) knots 0 0 0 1 2 2 2
  spline S187 degree 2 poles (6.8182, -15.7356) (6.9935, -15.6588) (7.1937, -15.4464) (7.251, -15.3) knots 0 0 0 1 2 2 2
  spline S188 degree 2 poles (7.251, -15.3) (7.3041, -15.152) (7.2957, -14.8557) (7.2368, -14.6827) knots 0 0 0 1 2 2 2
  line L164 (7.2368, -14.6827) -> (5.8538, -15.2883)
  spline S189 degree 2 poles (3.1319, -14.2016) (3.4201, -14.1322) (3.94, -14.1945) (4.1544, -14.3335) knots 0 0 0 1 2 2 2
  spline S190 degree 2 poles (4.1544, -14.3335) (4.3681, -14.4694) (4.6886, -14.9703) (4.7767, -15.3365) knots 0 0 0 1 2 2 2
  spline S191 degree 2 poles (4.7767, -15.3365) (4.8648, -15.7028) (4.7982, -16.284) (4.6765, -16.5039) knots 0 0 0 1 2 2 2
  spline S192 degree 2 poles (4.6765, -16.5039) (4.5554, -16.7267) (4.113, -17.0395) (3.8309, -17.1074) knots 0 0 0 1 2 2 2
  spline S193 degree 2 poles (3.8309, -17.1074) (3.6027, -17.1623) (3.1454, -17.1357) (2.9601, -17.0914) knots 0 0 0 1 2 2 2
  line L165 (2.9601, -17.0914) -> (2.8337, -16.566)
  line L166 (2.8337, -16.566) -> (2.8607, -16.5595)
  spline S194 degree 2 poles (2.8607, -16.5595) (2.9219, -16.5893) (3.104, -16.6598) (3.2287, -16.6901) knots 0 0 0 1 2 2 2
  spline S195 degree 2 poles (3.2287, -16.6901) (3.3394, -16.7143) (3.6216, -16.7258) (3.7417, -16.697) knots 0 0 0 1 2 2 2
  spline S196 degree 2 poles (3.7417, -16.697) (4.1049, -16.6096) (4.414, -15.9541) (4.2934, -15.4528) knots 0 0 0 1 2 2 2
  spline S197 degree 2 poles (4.2934, -15.4528) (4.1757, -14.9635) (3.6173, -14.5167) (3.2391, -14.6076) knots 0 0 0 1 2 2 2
  spline S198 degree 2 poles (3.2391, -14.6076) (3.0109, -14.6625) (2.6422, -14.9513) (2.5185, -15.1367) knots 0 0 0 1 2 2 2
  line L167 (2.5185, -15.1367) -> (2.4914, -15.1431)
  line L168 (2.4914, -15.1431) -> (2.3651, -14.6178)
  spline S199 degree 2 poles (2.3651, -14.6178) (2.4262, -14.5682) (2.6139, -14.4246) (2.6929, -14.3834) knots 0 0 0 1 2 2 2
  spline S200 degree 2 poles (2.6929, -14.3834) (2.8043, -14.3184) (2.9848, -14.2369) (3.1319, -14.2016) knots 0 0 0 1 2 2 2
  spline S201 degree 2 poles (0.6516, -14.5271) (1.3359, -14.4864) (2.1335, -15.2092) (2.1756, -15.918) knots 0 0 0 1 2 2 2
  spline S202 degree 2 poles (2.1756, -15.918) (2.217, -16.6146) (1.5357, -17.484) (0.947, -17.519) knots 0 0 0 1 2 2 2
  spline S203 degree 2 poles (0.947, -17.519) (0.682, -17.5348) (0.2629, -17.405) (0.1021, -17.2506) knots 0 0 0 1 2 2 2
  spline S204 degree 2 poles (0.1021, -17.2506) (-0.0617, -17.0964) (-0.253, -16.6346) (-0.2734, -16.2925) knots 0 0 0 1 2 2 2
  line L169 (-0.2734, -16.2925) -> (-0.289, -16.0305)
  line L170 (-0.289, -16.0305) -> (1.6867, -15.9131)
  spline S205 degree 2 poles (1.6867, -15.9131) (1.6572, -15.4169) (1.1265, -14.9195) (0.6827, -14.9459) knots 0 0 0 1 2 2 2
  spline S206 degree 2 poles (0.6827, -14.9459) (0.5255, -14.9552) (0.2246, -15.0443) (0.1046, -15.1071) knots 0 0 0 1 2 2 2
  spline S207 degree 2 poles (0.1046, -15.1071) (-0.0211, -15.1764) (-0.1935, -15.2949) (-0.2491, -15.3477) knots 0 0 0 1 2 2 2
  line L171 (-0.2491, -15.3477) -> (-0.2769, -15.3493)
  line L172 (-0.2769, -15.3493) -> (-0.308, -14.8254)
  spline S208 degree 2 poles (-0.308, -14.8254) (-0.2268, -14.7865) (0.0201, -14.6729) (0.117, -14.6393) knots 0 0 0 1 2 2 2
  spline S209 degree 2 poles (0.117, -14.6393) (0.2533, -14.591) (0.479, -14.5374) (0.6516, -14.5271) knots 0 0 0 1 2 2 2
  spline S210 degree 2 poles (0.2013, -16.3694) (0.219, -16.5632) (0.316, -16.842) (0.3987, -16.933) knots 0 0 0 1 2 2 2
  spline S211 degree 2 poles (0.3987, -16.933) (0.4884, -17.0359) (0.7571, -17.1344) (0.9513, -17.1228) knots 0 0 0 1 2 2 2
  spline S212 degree 2 poles (0.9513, -17.1228) (1.1424, -17.1115) (1.4038, -16.9815) (1.5081, -16.864) knots 0 0 0 1 2 2 2
  spline S213 degree 2 poles (1.5081, -16.864) (1.6092, -16.7435) (1.7039, -16.4626) (1.7085, -16.2798) knots 0 0 0 1 2 2 2
  line L173 (1.7085, -16.2798) -> (0.2013, -16.3694)
  spline S214 degree 2 poles (-9.4518, 2.9626) (-8.7462, 2.8397) (-8.0298, 2.0223) (-8.1194, 1.5083) knots 0 0 0 1 2 2 2
  spline S215 degree 2 poles (-8.1194, 1.5083) (-8.1559, 1.2984) (-8.3094, 0.9929) (-8.4389, 0.8431) knots 0 0 0 1 2 2 2
  line L174 (-8.4389, 0.8431) -> (-7.2587, 0.6376)
  line L175 (-7.2587, 0.6376) -> (-7.3414, 0.163)
  line L176 (-7.3414, 0.163) -> (-11.1953, 0.8343)
  line L177 (-11.1953, 0.8343) -> (-11.1126, 1.3088)
  line L178 (-11.1126, 1.3088) -> (-10.8176, 1.2574)
  spline S216 degree 2 poles (-10.8176, 1.2574) (-10.948, 1.4619) (-11.0857, 1.931) (-11.0418, 2.1834) knots 0 0 0 1 2 2 2
  spline S217 degree 2 poles (-11.0418, 2.1834) (-10.9575, 2.6671) (-10.0967, 3.075) (-9.4518, 2.9626) knots 0 0 0 1 2 2 2
  spline S218 degree 2 poles (-9.4824, 2.4634) (-9.966, 2.5476) (-10.5518, 2.3331) (-10.6117, 1.9894) knots 0 0 0 1 2 2 2
  spline S219 degree 2 poles (-10.6117, 1.9894) (-10.6467, 1.7887) (-10.5329, 1.3802) (-10.4221, 1.1886) knots 0 0 0 1 2 2 2
  line L179 (-10.4221, 1.1886) -> (-8.8222, 0.9099)
  spline S220 degree 2 poles (-8.8222, 0.9099) (-8.7017, 1.0801) (-8.5886, 1.333) (-8.559, 1.5034) knots 0 0 0 1 2 2 2
  spline S221 degree 2 poles (-8.559, 1.5034) (-8.4949, 1.8714) (-8.9653, 2.3733) (-9.4824, 2.4634) knots 0 0 0 1 2 2 2
  line L180 (-9.1831, 6.4926) -> (-7.1919, 4.1752)
  line L181 (-7.1919, 4.1752) -> (-7.3994, 3.796)
  line L182 (-7.3994, 3.796) -> (-10.4203, 4.2308)
  line L183 (-10.4203, 4.2308) -> (-10.1699, 4.6886)
  line L184 (-10.1699, 4.6886) -> (-7.8637, 4.3174)
  line L185 (-7.8637, 4.3174) -> (-9.4231, 6.0538)
  line L186 (-9.4231, 6.0538) -> (-9.1831, 6.4926)
  spline S222 degree 2 poles (-6.0255, 8.3424) (-5.331, 7.5884) (-5.1188, 6.4784) (-5.5753, 6.058) knots 0 0 0 1 2 2 2
  spline S223 degree 2 poles (-5.5753, 6.058) (-6.0386, 5.6313) (-7.1354, 5.9517) (-7.8152, 6.6898) knots 0 0 0 1 2 2 2
  spline S224 degree 2 poles (-7.8152, 6.6898) (-8.5139, 7.4483) (-8.7219, 8.5537) (-8.2631, 8.9763) knots 0 0 0 1 2 2 2
  spline S225 degree 2 poles (-8.2631, 8.9763) (-7.8021, 9.4009) (-6.699, 9.0736) (-6.0255, 8.3424) knots 0 0 0 1 2 2 2
  spline S226 degree 2 poles (-5.7205, 7.045) (-5.7936, 7.2338) (-6.1414, 7.7025) (-6.407, 7.991) knots 0 0 0 1 2 2 2
  spline S227 degree 2 poles (-6.407, 7.991) (-6.6727, 8.2794) (-7.1092, 8.6622) (-7.2978, 8.753) knots 0 0 0 1 2 2 2
  spline S228 degree 2 poles (-7.2978, 8.753) (-7.4863, 8.8438) (-7.8199, 8.8094) (-7.9766, 8.6651) knots 0 0 0 1 2 2 2
  spline S229 degree 2 poles (-7.9766, 8.6651) (-8.1333, 8.5208) (-8.1994, 8.187) (-8.1225, 7.985) knots 0 0 0 1 2 2 2
  spline S230 degree 2 poles (-8.1225, 7.985) (-8.0475, 7.7896) (-7.6868, 7.316) (-7.4337, 7.0412) knots 0 0 0 1 2 2 2
  spline S231 degree 2 poles (-7.4337, 7.0412) (-7.1618, 6.7459) (-6.7615, 6.3842) (-6.5602, 6.2842) knots 0 0 0 1 2 2 2
  spline S232 degree 2 poles (-6.5602, 6.2842) (-6.3718, 6.189) (-6.0254, 6.2185) (-5.8619, 6.3691) knots 0 0 0 1 2 2 2
  spline S233 degree 2 poles (-5.8619, 6.3691) (-5.7074, 6.5113) (-5.6413, 6.8451) (-5.7205, 7.045) knots 0 0 0 1 2 2 2
  spline S234 degree 2 poles (-4.7343, 10.7679) (-4.8621, 10.7133) (-5.0881, 10.5429) (-5.1896, 10.4425) knots 0 0 0 1 2 2 2
  spline S235 degree 2 poles (-5.1896, 10.4425) (-5.2825, 10.3457) (-5.4064, 10.1719) (-5.4523, 10.0986) knots 0 0 0 1 2 2 2
  line L187 (-5.4523, 10.0986) -> (-5.4806, 10.0865)
  line L188 (-5.4806, 10.0865) -> (-5.6929, 10.5834)
  spline S236 degree 2 poles (-5.6929, 10.5834) (-5.5748, 10.7312) (-5.1065, 11.089) (-4.8708, 11.1897) knots 0 0 0 1 2 2 2
  spline S237 degree 2 poles (-4.8708, 11.1897) (-4.6323, 11.2916) (-4.2362, 11.3467) (-4.0477, 11.3063) knots 0 0 0 1 2 2 2
  spline S238 degree 2 poles (-4.0477, 11.3063) (-3.8471, 11.2611) (-3.551, 11.0082) (-3.4588, 10.7924) knots 0 0 0 1 2 2 2
  spline S239 degree 2 poles (-3.4588, 10.7924) (-3.3351, 10.5028) (-3.5288, 9.903) (-3.7714, 9.7322) knots 0 0 0 1 2 2 2
  line L189 (-3.7714, 9.7322) -> (-3.7569, 9.6981)
  spline S240 degree 2 poles (-3.7569, 9.6981) (-3.6364, 9.7227) (-3.3401, 9.7284) (-3.1885, 9.6723) knots 0 0 0 1 2 2 2
  spline S241 degree 2 poles (-3.1885, 9.6723) (-3.0382, 9.619) (-2.766, 9.3593) (-2.6678, 9.1293) knots 0 0 0 1 2 2 2
  spline S242 degree 2 poles (-2.6678, 9.1293) (-2.5671, 8.8936) (-2.5579, 8.4241) (-2.6401, 8.2077) knots 0 0 0 1 2 2 2
  spline S243 degree 2 poles (-2.6401, 8.2077) (-2.7255, 7.9832) (-3.0895, 7.633) (-3.365, 7.5153) knots 0 0 0 1 2 2 2
  spline S244 degree 2 poles (-3.365, 7.5153) (-3.629, 7.4025) (-4.2003, 7.3095) (-4.414, 7.3224) knots 0 0 0 1 2 2 2
  line L190 (-4.414, 7.3224) -> (-4.6262, 7.8192)
  line L191 (-4.6262, 7.8192) -> (-4.5922, 7.8338)
  spline S245 degree 2 poles (-4.5922, 7.8338) (-4.3984, 7.789) (-3.8138, 7.8037) (-3.5668, 7.9092) knots 0 0 0 1 2 2 2
  spline S246 degree 2 poles (-3.5668, 7.9092) (-3.422, 7.9711) (-3.1712, 8.1857) (-3.1195, 8.332) knots 0 0 0 1 2 2 2
  spline S247 degree 2 poles (-3.1195, 8.332) (-3.0707, 8.477) (-3.0781, 8.7693) (-3.1594, 8.9596) knots 0 0 0 1 2 2 2
  spline S248 degree 2 poles (-3.1594, 8.9596) (-3.2406, 9.1498) (-3.4569, 9.3495) (-3.5866, 9.3781) knots 0 0 0 1 2 2 2
  spline S249 degree 2 poles (-3.5866, 9.3781) (-3.7163, 9.4066) (-4.0091, 9.3453) (-4.1681, 9.2774) knots 0 0 0 1 2 2 2
  line L192 (-4.1681, 9.2774) -> (-4.3668, 9.1925)
  line L193 (-4.3668, 9.1925) -> (-4.533, 9.5815)
  line L194 (-4.533, 9.5815) -> (-4.3768, 9.6482)
  spline S250 degree 2 poles (-4.3768, 9.6482) (-4.0617, 9.7828) (-3.7927, 10.2536) (-3.9152, 10.5403) knots 0 0 0 1 2 2 2
  spline S251 degree 2 poles (-3.9152, 10.5403) (-3.9722, 10.6738) (-4.1557, 10.8204) (-4.2623, 10.842) knots 0 0 0 1 2 2 2
  spline S252 degree 2 poles (-4.2623, 10.842) (-4.3758, 10.864) (-4.6122, 10.8201) (-4.7343, 10.7679) knots 0 0 0 1 2 2 2
  dimension "d9" = 33.02
  constraints: 1 centre point, 1 coincident, 1 other
  measures "d9" diameter of A0
emboss "Emboss1" sketch "Sketch4" operation cut depth 1.27 direction (0, 0, 1)
sketch "Sketch6" plane through (-3.6662, 6.35, 17.4625) normal (0, 1, 0) x (1, 0, 0)
  line L0 (7.3323, 0) -> (0, 0) construction
  line L1 (3.6662, 0) -> (3.6662, 34.6111) construction
  line L2 (16.1757, 34.925) -> (-8.8433, 34.925) projected
  point P0 (3.6662, 17.4625)
  point P1 (3.6662, 4.511)
  point P2 (3.6662, 28.7274)
  dimension "d12" = 4.511
  dimension "d13" = 6.1976
  constraints: 2 end point, 2 point on line, 1 midpoint, 1 vertical
  measures "d12" distance from line of point (3.666, 4.511) L0
  measures "d13" distance from line of point (3.666, 28.727) L2
hole "Hole1" at (0, 6.35, 12.9515) at (0, 6.35, -11.2649) direction (0, -1, 0) diameter 4.318 end through all clearance for "Hex Machine Screw" size "#6" standard "Ansi Unified Screw Threads"
equation "\"d0\" = printedHexSize"
equation "\"d1\" = length"
equation "\"d3\" = bushingDiameter"
equation "\"hexSize\" = 12.7"
equation "\"slipFitOffset\" = 0"
equation "\"printedHexSize\" = hexSize - slipFitOffset"
equation "\"length\" = 34.925"
equation "\"bushingSlipOffset\" = 0.381"
equation "\"bushingDiameter\" = 25.019"
body "Solid1"
